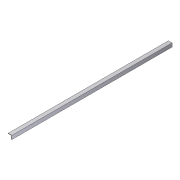
# Autodesk Inventor part: FE-00007-02
Saved by Autodesk Inventor 2012 (Build 160160000, 160)
## iProperties
Created: 2008-05-27
Part Number: FE-00007-02
Description: Lower Rail
Document SubType Name: Modeling
Designer: narosenberg
Density: 1 g/cm^3
Mass: 385.368 g
Surface Area: 2537.7 cm^2
Volume: 385.368 cm^3
Material: Default
Author: narosenberg
Autodesk Inventor part; units mm, degrees
ref_plane "YZ Plane" through (0, 0, 0) normal (1, 0, 0) x (0, 1, 0)
ref_plane "XZ Plane" through (0, 0, 0) normal (0, 1, 0) x (-1, 0, 0)
ref_plane "XY Plane" through (0, 0, 0) normal (0, 0, 1) x (1, 0, 0)
sketch "Sketch1" plane through (0, 0, 0) normal (0, 0, 1) x (1, 0, 0)
  line L0 (-31.6692, 26.6271) -> (6.4308, 26.6271)
  line L1 (6.4308, 26.6271) -> (6.4308, -11.4729)
  line L2 (6.4308, -11.4729) -> (3.2558, -11.4729)
  line L3 (-31.6692, 23.4521) -> (-31.6692, 26.6271)
  line L4 (-31.6692, 23.4521) -> (3.2558, 23.4521)
  line L5 (3.2558, 23.4521) -> (3.2558, -11.4729)
  dimension "d0" = 38.1
  dimension "d1" = 38.1
  dimension "d2" = 3.175
  dimension "d3" = 3.175
  constraints: 12 end point, 2 horizontal, 2 parallel, 2 perpendicular
  measures "d0" distance of L0.start L0.end
  measures "d1" distance of L0.end L1.end
  measures "d2" distance of L3.start L0.start
  measures "d3" distance of L1.end L2.end
extrude "Extrusion1" add sketch "Sketch1" along normal blind 1662.1125
body "Solid1"
